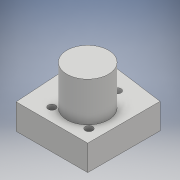
# Autodesk Inventor part: Cover
Saved by Autodesk Inventor 2017 (Build 210142000, 142)
## iProperties
Created: 2018-01-31
Part Number: Cover
Material: Generic
Document SubType Name: Modeling
Designer: andrew
Density: 1 g/cm^3
Appearance: Default
Author: andrew
Autodesk Inventor part; units mm, degrees
ref_plane "YZ Plane" through (0, 0, 0) normal (1, 0, 0) x (0, 1, 0)
ref_plane "XZ Plane" through (0, 0, 0) normal (0, 1, 0) x (-1, 0, 0)
ref_plane "XY Plane" through (0, 0, 0) normal (0, 0, 1) x (1, 0, 0)
sketch "Sketch1" plane through (0, 0, 0) normal (0, 0, 1) x (1, 0, 0)
  line L0 (-2.8403, 5.136) -> (-4.6718, 3.4343)
  line L1 (-4.2463, -3.182) -> (-4.6718, 3.4343)
  line L2 (-4.2463, -3.182) -> (3.182, -3.182)
  line L3 (3.182, -3.182) -> (3.182, 4.3178)
  line L4 (-2.8403, 5.136) -> (3.182, 4.3178)
  circle A0 centre (0, 0) radius 1.2484
  circle A1 centre (0, 3) radius 0.7934
  circle A2 centre (-1.875, -1.75) radius 0.7934
  circle A3 centre (1.875, -1.75) radius 0.7934
  line L5 (-4.569, 3.3933) -> (-2.8069, 5.0305)
  line L6 (-2.8069, 5.0305) -> (3.082, 4.2305)
  line L7 (3.082, 4.2305) -> (3.082, -3.082)
  line L8 (3.082, -3.082) -> (-4.1525, -3.082)
  line L9 (-4.1525, -3.082) -> (-4.569, 3.3933)
  dimension "d0" = 0.1
  constraints: 20 end point, 4 centre point, 4 other
  measures "d0" distance between parallel lines of L0 L5
extrude "Extrusion1" add sketch "Sketch1" along normal blind 1 contours L5 L6 L7 L8 L9
sketch "Sketch2" plane through (0, 0, 1) normal (0, 0, 1) x (1, 0, 0)
  line L0 (-2.8403, 5.136) -> (-4.6718, 3.4343)
  line L1 (-4.2463, -3.182) -> (-4.6718, 3.4343)
  line L2 (-4.2463, -3.182) -> (3.182, -3.182)
  line L3 (3.182, -3.182) -> (3.182, 4.3178)
  line L4 (-2.8403, 5.136) -> (3.182, 4.3178)
  circle A0 centre (0, 0) radius 1.2484
  circle A1 centre (0, 3) radius 0.7934
  circle A2 centre (-1.875, -1.75) radius 0.7934
  circle A3 centre (1.875, -1.75) radius 0.7934
  line L5 (-4.569, 3.3933) -> (-2.8069, 5.0305)
  line L6 (-2.8069, 5.0305) -> (3.082, 4.2305)
  line L7 (3.082, 4.2305) -> (3.082, -3.082)
  line L8 (3.082, -3.082) -> (-4.1525, -3.082)
  line L9 (-4.1525, -3.082) -> (-4.569, 3.3933)
  circle A4 centre (0, 3) radius 0.375
  circle A5 centre (1.875, -1.75) radius 0.375
  circle A6 centre (-1.875, -1.75) radius 0.375
  dimension "d3" = 0.1
  dimension "d4" = 1.5869
  dimension "d5" = 0.75
  dimension "d6" = 0.75
  dimension "d7" = 0.75
  constraints: 20 end point, 7 centre point, 3 coincident, 4 other
  measures "d3" distance between parallel lines of L0 L5
  measures "d4" diameter of A1
  measures "d5" diameter of A4
  measures "d6" diameter of A5
  measures "d7" diameter of A6
extrude "Extrusion2" add sketch "Sketch2" along normal blind 4.43 contours A1 | A2 | A3 | L5 L6 L7 L8 L9
sketch "Sketch3" plane through (0, 0, 5.43) normal (0, 0, 1) x (1, 0, 0)
  line L0 (-2.8403, 5.136) -> (-4.6718, 3.4343)
  line L1 (-4.2463, -3.182) -> (-4.6718, 3.4343)
  line L2 (-4.2463, -3.182) -> (3.182, -3.182)
  line L3 (3.182, -3.182) -> (3.182, 4.3178)
  line L4 (-2.8403, 5.136) -> (3.182, 4.3178)
  circle A0 centre (0, 0) radius 1.2484
  circle A1 centre (0, 3) radius 0.7934
  circle A2 centre (-1.875, -1.75) radius 0.7934
  circle A3 centre (1.875, -1.75) radius 0.7934
  line L5 (-4.569, 3.3933) -> (-2.8069, 5.0305)
  line L6 (-2.8069, 5.0305) -> (3.082, 4.2305)
  line L7 (3.082, 4.2305) -> (3.082, -3.082)
  line L8 (3.082, -3.082) -> (-4.1525, -3.082)
  line L9 (-4.1525, -3.082) -> (-4.569, 3.3933)
  circle A4 centre (0, 3) radius 0.375
  circle A5 centre (1.875, -1.75) radius 0.375
  circle A6 centre (-1.875, -1.75) radius 0.375
  dimension "d10" = 0.1
  dimension "d11" = 1.5869
  dimension "d12" = 0.75
  dimension "d13" = 0.75
  dimension "d14" = 0.75
  constraints: 20 end point, 7 centre point, 3 coincident, 4 other
  measures "d10" distance between parallel lines of L0 L5
  measures "d11" diameter of A1
  measures "d12" diameter of A4
  measures "d13" diameter of A5
  measures "d14" diameter of A6
extrude "Extrusion3" add sketch "Sketch3" along normal blind 1 contours A0 | A1 | A2 | A3 | L5 L6 L7 L8 L9
sketch "Sketch5" plane through (0, 0, 6.43) normal (0, 0, 1) x (1, 0, 0)
  circle A0 centre (0, 0) radius 1.2484 projected
  circle A1 centre (0, 0) radius 2.1
  line L0 (5.5495, -5.5229) -> (-7.4793, -5.5229)
  line L1 (-7.4793, -5.5229) -> (-7.4793, 6.9136)
  line L2 (-7.4793, 6.9136) -> (5.5495, 6.9136)
  line L3 (5.5495, 6.9136) -> (5.5495, -5.5229)
  dimension "d18" = 4.2
  constraints: 8 end point, 2 parallel, 1 centre point, 1 coincident, 1 horizontal, 1 perpendicular
  measures "d18" diameter of A1
extrude "Extrusion4" cut sketch "Sketch5" against normal blind 4 contours L0 L1 L2 L3
sketch "Sketch6" plane through (0, 0, 0) normal (0, 0, -1) x (-1, 0, 0)
  circle A0 centre (0, 0) radius 1.2484 projected
  circle A1 centre (0, 3) radius 0.7934 projected
  circle A2 centre (1.875, -1.75) radius 0.7934 projected
  circle A3 centre (-1.875, -1.75) radius 0.7934 projected
  line L0 (4.569, 3.3933) -> (2.8069, 5.0305) projected
  line L1 (2.8069, 5.0305) -> (-3.082, 4.2305) projected
  line L2 (-3.082, 4.2305) -> (-3.082, -3.082) projected
  line L3 (-3.082, -3.082) -> (4.1525, -3.082) projected
  line L4 (4.1525, -3.082) -> (4.569, 3.3933) projected
extrude "Extrusion5" add sketch "Sketch6" along normal blind 0.15
chamfer "Chamfer1" distance 0.2 angle 45 4 edges at (-1.0816, -1.75, -0.15) (2.6684, -1.75, -0.15) (0.7934, 3, -0.15) (1.2484, 0, -0.15)
body "Solid1"
